Autodesk Inventor part; units mm, degrees
(part 2 of 2)
  circle A449 centre (92.8688, -61.9125) radius 1.994
  circle A450 centre (87.7887, -61.9125) radius 0.851
  circle A451 centre (97.9488, -61.9125) radius 0.851
  circle A452 centre (164.3063, -42.8625) radius 1.994
  circle A453 centre (159.2262, -42.8625) radius 0.851
  circle A454 centre (169.3862, -42.8625) radius 0.851
  circle A455 centre (173.8313, -61.9125) radius 1.994
  circle A456 centre (168.7512, -61.9125) radius 0.851
  circle A457 centre (178.9112, -61.9125) radius 0.851
  circle A458 centre (178.5938, -80.9625) radius 1.994
  circle A459 centre (173.5138, -80.9625) radius 0.851
  circle A460 centre (183.6738, -80.9625) radius 0.851
  circle A461 centre (188.1188, -100.0125) radius 1.994
  circle A462 centre (183.0388, -100.0125) radius 0.851
  circle A463 centre (193.1987, -100.0125) radius 0.851
  circle A464 centre (183.3562, -42.8625) radius 1.994
  circle A465 centre (178.2763, -42.8625) radius 0.851
  circle A466 centre (188.4363, -42.8625) radius 0.851
  circle A467 centre (192.8813, -61.9125) radius 1.994
  circle A468 centre (187.8013, -61.9125) radius 0.851
  circle A469 centre (197.9613, -61.9125) radius 0.851
  circle A470 centre (197.6438, -80.9625) radius 1.994
  circle A471 centre (192.5638, -80.9625) radius 0.851
  circle A472 centre (202.7237, -80.9625) radius 0.851
  circle A473 centre (207.1688, -100.0125) radius 1.994
  circle A474 centre (202.0888, -100.0125) radius 0.851
  circle A475 centre (212.2488, -100.0125) radius 0.851
  circle A476 centre (95.25, -80.9625) radius 1.994
  circle A477 centre (90.17, -80.9625) radius 0.851
  circle A478 centre (100.33, -80.9625) radius 0.851
  circle A479 centre (202.4062, -42.8625) radius 1.994
  circle A480 centre (197.3262, -42.8625) radius 0.851
  circle A481 centre (207.4863, -42.8625) radius 0.851
  circle A482 centre (211.9313, -61.9125) radius 1.994
  circle A483 centre (206.8512, -61.9125) radius 0.851
  circle A484 centre (217.0113, -61.9125) radius 0.851
  circle A485 centre (216.6938, -80.9625) radius 1.994
  circle A486 centre (211.6138, -80.9625) radius 0.851
  circle A487 centre (221.7738, -80.9625) radius 0.851
  circle A488 centre (226.2188, -100.0125) radius 1.994
  circle A489 centre (221.1388, -100.0125) radius 0.851
  circle A490 centre (231.2988, -100.0125) radius 0.851
  circle A491 centre (209.55, -119.0625) radius 1.994
  circle A492 centre (204.47, -119.0625) radius 0.851
  circle A493 centre (214.63, -119.0625) radius 0.851
  circle A494 centre (159.512, -112.0775) radius 1.524
  circle A495 centre (259.588, -112.0775) radius 1.524
  circle A496 centre (159.512, -127.3175) radius 1.994
  circle A497 centre (259.588, -127.3175) radius 1.994
  circle A498 centre (221.4563, -42.8625) radius 1.994
  circle A499 centre (216.3762, -42.8625) radius 0.851
  circle A500 centre (226.5363, -42.8625) radius 0.851
  circle A501 centre (230.9812, -61.9125) radius 1.994
  circle A502 centre (225.9013, -61.9125) radius 0.851
  circle A503 centre (236.0613, -61.9125) radius 0.851
  circle A504 centre (235.7438, -80.9625) radius 1.994
  circle A505 centre (230.6637, -80.9625) radius 0.851
  circle A506 centre (240.8237, -80.9625) radius 0.851
  circle A507 centre (245.2688, -100.0125) radius 1.994
  circle A508 centre (240.1888, -100.0125) radius 0.851
  circle A509 centre (250.3487, -100.0125) radius 0.851
  circle A510 centre (100.0125, -100.0125) radius 1.994
  circle A511 centre (94.9325, -100.0125) radius 0.851
  circle A512 centre (105.0925, -100.0125) radius 0.851
  circle A513 centre (88.0745, -93.0275) radius 1.524
  circle A514 centre (111.9505, -93.0275) radius 1.524
  circle A515 centre (88.0745, -108.2675) radius 1.994
  circle A516 centre (111.9505, -108.2675) radius 1.994
  circle A517 centre (240.5062, -42.8625) radius 1.994
  circle A518 centre (235.4263, -42.8625) radius 0.851
  circle A519 centre (245.5863, -42.8625) radius 0.851
  circle A520 centre (250.0312, -61.9125) radius 1.994
  circle A521 centre (244.9513, -61.9125) radius 0.851
  circle A522 centre (255.1113, -61.9125) radius 0.851
  circle A523 centre (254.7938, -80.9625) radius 1.994
  circle A524 centre (249.7138, -80.9625) radius 0.851
  circle A525 centre (259.8737, -80.9625) radius 0.851
  circle A526 centre (264.3188, -100.0125) radius 1.994
  circle A527 centre (259.2387, -100.0125) radius 0.851
  circle A528 centre (269.3988, -100.0125) radius 0.851
  circle A529 centre (259.5562, -42.8625) radius 1.994
  circle A530 centre (254.4763, -42.8625) radius 0.851
  circle A531 centre (264.6363, -42.8625) radius 0.851
  circle A532 centre (269.0813, -61.9125) radius 1.994
  circle A533 centre (264.0013, -61.9125) radius 0.851
  circle A534 centre (274.1612, -61.9125) radius 0.851
  circle A535 centre (273.8438, -80.9625) radius 1.994
  circle A536 centre (268.7638, -80.9625) radius 0.851
  circle A537 centre (278.9238, -80.9625) radius 0.851
  circle A538 centre (283.3687, -100.0125) radius 1.994
  circle A539 centre (278.2887, -100.0125) radius 0.851
  circle A540 centre (288.4488, -100.0125) radius 0.851
  circle A541 centre (90.4875, -119.0625) radius 1.994
  circle A542 centre (85.4075, -119.0625) radius 0.851
  circle A543 centre (95.5675, -119.0625) radius 0.851
  circle A544 centre (278.6062, -42.8625) radius 1.994
  circle A545 centre (273.5263, -42.8625) radius 0.851
  circle A546 centre (283.6862, -42.8625) radius 0.851
  circle A547 centre (288.1313, -61.9125) radius 1.994
  circle A548 centre (283.0512, -61.9125) radius 0.851
  circle A549 centre (293.2113, -61.9125) radius 0.851
  circle A550 centre (292.8938, -80.9625) radius 1.994
  circle A551 centre (287.8138, -80.9625) radius 0.851
  circle A552 centre (297.9737, -80.9625) radius 0.851
  circle A553 centre (302.4187, -100.0125) radius 1.994
  circle A554 centre (297.3388, -100.0125) radius 0.851
  circle A555 centre (307.4987, -100.0125) radius 0.851
  circle A556 centre (278.6062, -119.0625) radius 1.994
  circle A557 centre (273.5263, -119.0625) radius 0.851
  circle A558 centre (283.6862, -119.0625) radius 0.851
  circle A559 centre (297.6562, -42.8625) radius 1.994
  circle A560 centre (292.5763, -42.8625) radius 0.851
  circle A561 centre (302.7362, -42.8625) radius 0.851
  circle A562 centre (307.1812, -61.9125) radius 1.994
  circle A563 centre (302.1012, -61.9125) radius 0.851
  circle A564 centre (312.2613, -61.9125) radius 0.851
  circle A565 centre (311.9438, -80.9625) radius 1.994
  circle A566 centre (306.8637, -80.9625) radius 0.851
  circle A567 centre (317.0238, -80.9625) radius 0.851
  circle A568 centre (328.6125, -100.0125) radius 1.994
  circle A569 centre (323.5325, -100.0125) radius 0.851
  circle A570 centre (333.6925, -100.0125) radius 0.851
  circle A571 centre (107.1563, -42.8625) radius 1.994
  circle A572 centre (102.0763, -42.8625) radius 0.851
  circle A573 centre (112.2362, -42.8625) radius 0.851
  circle A574 centre (297.6562, -119.0625) radius 1.994
  circle A575 centre (292.5763, -119.0625) radius 0.851
  circle A576 centre (302.7362, -119.0625) radius 0.851
  circle A577 centre (316.7063, -42.8625) radius 1.994
  circle A578 centre (311.6263, -42.8625) radius 0.851
  circle A579 centre (321.7863, -42.8625) radius 0.851
  circle A580 centre (326.2313, -61.9125) radius 1.994
  circle A581 centre (321.1513, -61.9125) radius 0.851
  circle A582 centre (331.3112, -61.9125) radius 0.851
  circle A583 centre (342.9, -80.9625) radius 1.994
  circle A584 centre (337.82, -80.9625) radius 0.851
  circle A585 centre (347.98, -80.9625) radius 0.851
  circle A586 centre (330.962, -73.9775) radius 1.524
  circle A587 centre (354.838, -73.9775) radius 1.524
  circle A588 centre (330.962, -89.2175) radius 1.994
  circle A589 centre (354.838, -89.2175) radius 1.994
  circle A590 centre (354.8062, -100.0125) radius 1.994
  circle A591 centre (349.7262, -100.0125) radius 0.851
  circle A592 centre (359.8863, -100.0125) radius 0.851
  circle A593 centre (316.7063, -119.0625) radius 1.994
  circle A594 centre (311.6263, -119.0625) radius 0.851
  circle A595 centre (321.7863, -119.0625) radius 0.851
  circle A596 centre (345.2812, -42.8625) radius 1.994
  circle A597 centre (340.2013, -42.8625) radius 0.851
  circle A598 centre (350.3612, -42.8625) radius 0.851
  circle A599 centre (333.3433, -35.8775) radius 1.524
  circle A600 centre (357.2192, -35.8775) radius 1.524
  circle A601 centre (333.3433, -51.1175) radius 1.994
  circle A602 centre (357.2192, -51.1175) radius 1.994
  circle A603 centre (350.0438, -61.9125) radius 1.994
  circle A604 centre (344.9638, -61.9125) radius 0.851
  circle A605 centre (355.1237, -61.9125) radius 0.851
  circle A606 centre (373.8562, -80.9625) radius 1.994
  circle A607 centre (368.7763, -80.9625) radius 0.851
  circle A608 centre (378.9362, -80.9625) radius 0.851
  circle A609 centre (373.8562, -100.0125) radius 1.994
  circle A610 centre (368.7763, -100.0125) radius 0.851
  circle A611 centre (378.9362, -100.0125) radius 0.851
  circle A612 centre (116.6813, -61.9125) radius 1.994
  circle A613 centre (111.6013, -61.9125) radius 0.851
  circle A614 centre (121.7613, -61.9125) radius 0.851
  circle A615 centre (354.8062, -119.0625) radius 1.994
  circle A616 centre (349.7262, -119.0625) radius 0.851
  circle A617 centre (359.8863, -119.0625) radius 0.851
  circle A618 centre (373.8562, -42.8625) radius 1.994
  circle A619 centre (368.7763, -42.8625) radius 0.851
  circle A620 centre (378.9362, -42.8625) radius 0.851
  circle A621 centre (373.8562, -61.9125) radius 1.994
  circle A622 centre (368.7763, -61.9125) radius 0.851
  circle A623 centre (378.9362, -61.9125) radius 0.851
  circle A624 centre (335.7563, -119.0625) radius 1.994
  circle A625 centre (330.6762, -119.0625) radius 0.851
  circle A626 centre (340.8363, -119.0625) radius 0.851
  circle A627 centre (373.8562, -119.0625) radius 1.994
  circle A628 centre (368.7763, -119.0625) radius 0.851
  circle A629 centre (378.9362, -119.0625) radius 0.851
  circle A630 centre (121.4437, -80.9625) radius 1.994
  circle A631 centre (116.3638, -80.9625) radius 0.851
  circle A632 centre (126.5238, -80.9625) radius 0.851
  circle A633 centre (130.9688, -100.0125) radius 1.994
  circle A634 centre (125.8888, -100.0125) radius 0.851
  circle A635 centre (136.0488, -100.0125) radius 0.851
  constraints: 636 centre point, 560 end point, 560 point on circle
extrude "60pc_pcb.kicad_pcb_Outline" add sketch "Sketch1" along normal blind 1.6
body "Solid1"
